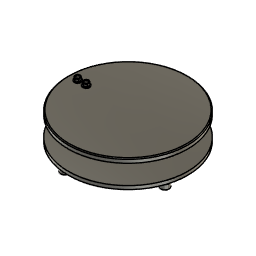
Wägezelle v2 (Autodesk Fusion 360 archive; units mm, degrees)
design "Wägezelle" references "Sechskantschraube mit Flansch und Vertiefung ANSI B18.6.7M - M4x0.7 x 16 Stahlklasse 2 Einfach", "Sechskantschraube mit Flansch und Vertiefung ANSI B18.6.7M - M4x0.7 x 20 Stahlklasse 2 Einfach"
Autodesk Fusion 360 part; units mm, degrees
note: some values were not read from the file. Chosen so that the rebuilt part matches the saved one: which bodies a step acts on; which face or edge a step refers to; how an offset face is resized. Set by a fixed rule: which sketch regions a step uses.
sketch "Skizze1" plane through (0, 0, 0) normal (0, 0, 1) x (1, 0, 0)
  line L0 (37.5, -6.35) -> (-37.5, -6.35)
  line L1 (-37.5, -6.35) -> (-37.5, 6.35)
  line L2 (-37.5, 6.35) -> (37.5, 6.35)
  line L3 (37.5, 6.35) -> (37.5, -6.35)
  line L4 (37.5, -6.35) -> (-37.5, 6.35) construction
  line L5 (-37.5, -6.35) -> (37.5, 6.35) construction
  dimension "d1" = 75
  dimension "d2" = 12.7
  constraint horizontal L0
  constraint perpendicular L0 L1
  constraint parallel L0 L2
  constraint parallel L1 L3
  constraint coincident L4 origin
  constraint coincident L5 origin
  measures "d1" distance of L1.end L2.end
  measures "d2" distance of L0.end L1.end
extrude "Extrusion1" add sketch "Skizze1" along normal blind 12.7 makes body 1
sketch "Skizze2" plane through (0, 0, 12.7) normal (0, 0, 1) x (-1, 0, 0)
  line L0 (-37.5, -6.35) -> (37.5, -6.35)
  line L1 (37.5, -6.35) -> (37.5, 6.35)
  line L2 (37.5, 6.35) -> (-37.5, 6.35)
  line L3 (-37.5, 6.35) -> (-37.5, -6.35)
  circle A0 centre (32, 0) radius 1.9
  circle A1 centre (22, 0) radius 1.9
  circle A2 centre (-32, 0) radius 1.9
  circle A3 centre (-22, 0) radius 1.9
  dimension "d8" = 3.8
  dimension "d9" = 3.8
  dimension "d10" = 5.5
  dimension "d11" = 15.5
  dimension "d12" = 3.8
  dimension "d13" = 3.8
  dimension "d14" = 5.5
  dimension "d15" = 15.5
  measures "d8" diameter of A0
  measures "d9" diameter of A1
  measures "d10" distance of L1 A0.centre
  measures "d11" distance of L1 A1.centre
  measures "d12" diameter of A2
  measures "d13" diameter of A3
  measures "d14" distance of L3 A2.centre
  measures "d15" distance of L3 A3.centre
extrude "Extrusion3" cut sketch "Skizze2" against normal through all contours A0 | A1 | A2 | A3 bodies 1
thread "Gewinde2" "ISO Metric profile 4.0 M4x0.7 6H" major diameter 4.1095 minor diameter 3.332 pitch 0.7 angle 60 resizes the face on face at (-33.8906, 0.1892, 4.2333) on bodies 1
thread "Gewinde3" "ISO Metric profile 4.0 M4x0.7 6H" major diameter 4.1095 minor diameter 3.332 pitch 0.7 angle 60 resizes the face on face at (-23.8906, 0.1892, 4.2333) on bodies 1
thread "Gewinde4" "ISO Metric profile 4.0 M4x0.7 6H" major diameter 4.1095 minor diameter 3.332 pitch 0.7 angle 60 resizes the face on face at (20.1094, 0.1892, 4.2333) on bodies 1
thread "Gewinde5" "ISO Metric profile 4.0 M4x0.7 6H" major diameter 4.1095 minor diameter 3.332 pitch 0.7 angle 60 resizes the face on face at (30.1094, 0.1892, 4.2333) on bodies 1
chamfer "Fase1" distance 0.5 angle 45 4 edges at (-37.5, 0, 12.7) (0, -6.35, 12.7) (0, 6.35, 12.7) (37.5, 0, 12.7) on bodies 1
chamfer "Fase2" distance 0.5 angle 45 1 edges at (37.5, 0, 0) 1 faces at (-7.2098, -4.7747, 0) on bodies 1
copy_body "Körper->Berechn2" bodies 1 removing the originals makes body 2 in component "Component'"
sketch "Skizze6" plane through (0, 0, 0) normal (0, 0, 1) x (1, 0, 0)
  line L0 (37, 5.85) -> (-37, 5.85)
  circle A0 centre (22, 0) radius 1.666
  circle A1 centre (32, 0) radius 1.666
  line L1 (-37, -5.85) -> (37, -5.85)
  line L2 (37, -5.85) -> (37, 5.85)
  line L3 (17.5276, 5.85) -> (37, 5.85)
  line L4 (37, 5.85) -> (37, -5.85)
  line L5 (37, -5.85) -> (17.5276, -5.85)
  line L6 (17.5276, -5.85) -> (17.5276, 5.85)
  circle A2 centre (32, 0) radius 1.9
  circle A3 centre (22, 0) radius 1.9
  dimension "d48" = 3.8
  dimension "d49" = 3.8
  constraint horizontal L3
  constraint vertical L4
  constraint horizontal L5
  constraint vertical L6
  constraint coincident L1.end L2.start
  constraint coincident L0 L3.start
  constraint concentric A1 A2
  constraint concentric A0 A3
  measures "d48" diameter of A2
  measures "d49" diameter of A3
extrude "Extrusion1'" add sketch "Skizze6" against normal blind 5 separate body contours L0 L1 L2 L3 L4 L5 L6 makes body 3 in component "Component'"
sketch "Skizze7" plane through (0, 0, -5) normal (0, 0, -1) x (1, 0, 0)
  circle A0 centre (32, 0) radius 1.9
  circle A1 centre (22, 0) radius 1.9
  line L0 (37, 5.85) -> (17.5276, 5.85)
  line L1 (17.5276, 5.85) -> (17.5276, -5.85)
  line L2 (17.5276, -5.85) -> (37, -5.85)
  line L3 (37, -5.85) -> (37, 5.85)
  circle A2 centre (26.9941, 0) radius 70
  dimension "d52" = 140
  measures "d52" diameter of A2
extrude "Extrusion2" add sketch "Skizze7" along normal blind 4 contours L0 L1 L2 L3 | A2 bodies 2 3 in component "Component'"
sketch "Skizze8" plane through (0, 0, -9) normal (0, 0, -1) x (1, 0, 0)
  circle A0 centre (32, 0) radius 1.9
  circle A1 centre (22, 0) radius 1.9
  circle A2 centre (26.9941, 0) radius 70
  circle A3 centre (42.3799, -58.7295) radius 5
  dimension "d55" = 10
  measures "d55" diameter of A3
extrude "Extrusion3'" add sketch "Skizze8" along normal blind 10 contours A3 bodies 3 in component "Component'"
fillet "Abrundung1" radius 4 1 edges at (37.7183, 56.9214, -9) on bodies 3 in component "Component'"
chamfer "Fase1'" distance 0.8 angle 45 1 edges at (37.7183, 60.5376, -19) on bodies 3 in component "Component'"
pattern_circular "C-Anordnung1" count 4 over 360 about axis through (26.9941, 0, -9) along (0, 0, -1) of "Extrusion3'" in component "Component'"
fillet "Abrundung2" radius 4 3 edges at (16.2698, -56.9214, -9) (-29.9274, 10.7242, -9) (83.9155, -10.7242, -9) on bodies 3 in component "Component'"
chamfer "Fase2'" distance 0.8 angle 45 3 edges at (87.5317, -10.7242, -19) (16.2698, -60.5376, -19) (-33.5435, 10.7242, -19) on bodies 3 in component "Component'"
sketch "Skizze9" plane through (0, 0, 12.7) normal (0, 0, 1) x (-1, 0, 0)
  circle A0 centre (32, 0) radius 1.666
  circle A1 centre (-32, 0) radius 1.666
  circle A2 centre (22, 0) radius 1.666
  circle A3 centre (-22, 0) radius 1.666
  line L0 (-37, 5.85) -> (-37, -5.85)
  line L1 (-37, -5.85) -> (37, -5.85)
  line L2 (37, -5.85) -> (37, 5.85)
  line L3 (37, 5.85) -> (-37, 5.85)
  circle A4 centre (22, 0) radius 1.666
  circle A5 centre (32, 0) radius 1.666
  line L4 (37, -5.85) -> (-37, -5.85)
  line L5 (37, 5.85) -> (37, -5.85)
  line L6 (-37, 5.85) -> (37, 5.85)
  line L7 (37, 5.85) -> (16.4735, 5.85)
  line L8 (16.4735, 5.85) -> (16.4735, -5.85)
  line L9 (16.4735, -5.85) -> (37, -5.85)
  line L10 (37, -5.85) -> (37, 5.85)
  constraint horizontal L7
  constraint vertical L8
  constraint horizontal L9
  constraint vertical L10
  constraint coincident L1 L8.end
  constraint coincident L2.end L3.start
extrude "Extrusion4" add sketch "Skizze9" along normal blind 5 separate body contours L1 L2 L3 L4 L5 L6 L7 L8 L9 L10 makes body 5 in component "Component'"
sketch "Skizze10" plane through (0, 0, 17.7) normal (0, 0, 1) x (-1, 0, 0)
  circle A0 centre (32, 0) radius 1.666
  circle A1 centre (22, 0) radius 1.666
  line L0 (37, -5.85) -> (37, 5.85)
  line L1 (37, 5.85) -> (16.4735, 5.85)
  line L2 (16.4735, 5.85) -> (16.4735, -5.85)
  line L3 (16.4735, -5.85) -> (37, -5.85)
  circle A2 centre (-26.9941, 0) radius 70
  circle A3 centre (-26.9941, 0) radius 70
  dimension "d68" = 140
  constraint concentric A2 A3
  measures "d68" diameter of A3
extrude "Extrusion4'" add sketch "Skizze10" along normal blind 5 separate body contours L0 L1 L2 L3 | A2 A3 makes body 6
other "Schraube1"
other "Schraube2"
chamfer "Fase3" distance 1 angle 45 1 edges at (92.257, 25.3131, 22.7) on bodies 6
component "Component'" placed x (1, 0, 0) y (0, 1, 0) z (0, 0, 1) at (0, 0, 0)
component "Wägezelle v2" placed x (1, 0, 0) y (0, 1, 0) z (0, 0, 1) at (0, 0, 0)
component "Wägezelle v2" placed x (1, 0, 0) y (0, 1, 0) z (0, 0, 1) at (0, 0, 0)

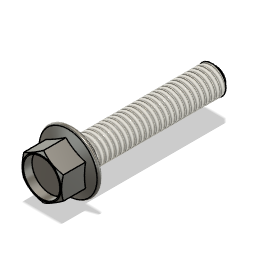
design "Sechskantschraube mit Flansch und Vertiefung ANSI B18.6.7M - M4x0.7 x 20 Stahlklasse 2 Einfach"
description: Sechskantschraube mit Flansch und Vertiefung ANSI B18.6.7M - M4x0.7 x 20
part number: IHFHMS ANSI B18.6.7M - M4x0.7 x 20 Stahlklasse 2 Einfach
Autodesk Fusion 360 part; units mm, degrees
sketch "Sketch1" plane through (0, 0, 0) normal (0, 1, 0) x (1, 0, 0)
  line L0 (-2, 0) -> (-2, 20)
  line L1 (-2, 20) -> (0, 20)
  line L2 (0, 20) -> (0, -3.1)
  line L3 (-2, 0) -> (-3.1763, 0)
  line L4 (-3.1763, 0) -> (-3.1763, -4.0222)
  line L5 (-2.695, -4.3) -> (-2.55, -4.3)
  line L6 (-2.695, -4.3) -> (-3.1763, -4.0222)
  line L7 (-2.55, -4.3) -> (-2.55, -3.1)
  line L8 (-2.55, -3.1) -> (0, -3.1)
  dimension "d9" = 4
  dimension "d111" = 4.3
  dimension "d113" = 30
  dimension "d114" = 6.3525
  dimension "d115" = 5.39
  dimension "d158" = 5.1
  dimension "d168" = 20
  dimension "d169" = 1.2
  constraint perpendicular L0 L1
  constraint perpendicular L0 L3
  constraint coincident origin L3
  constraint vertical L0
  constraint vertical L2
  constraint parallel L2 L4
  constraint coincident L2 L8.end
  constraint perpendicular L2 L5
  constraint coincident L3.end L4.start
  constraint perpendicular L5 L7
  constraint perpendicular L2 L8
  constraint coincident L2.end L8.end
  constraint coincident origin L2
  measures "d111" distance of L3 L5
  measures "d113" angle of L5 L6
  measures "d168" distance of origin L1
  measures "d169" distance of L5.end L8
revolve "Revolve1" add sketch "Sketch1" angle 360 about axis through (0, 0, -20) along (0, 0, 1)
sketch "Sketch8" plane through (0, 0, 0) normal (0, 0, 1) x (1, 0, 0)
  line L0 (0, 0) -> (-2.75, 0) construction
  line L1 (-2.75, -1.5894) -> (-2.75, 1.5894)
  circle A0 centre (0, 0) radius 3.1763
  dimension "d110" = 2.75
  constraint horizontal L0
  constraint perpendicular L0 L1
  constraint coincident L0.end L1
  constraint coincident L0.start A0.centre
  constraint coincident L1.end A0
  constraint coincident L1.start A0
  measures "d110" distance of L0.start L1
extrude "Extrude5" cut sketch "Sketch8" along normal blind 4.3 contours L1 A0 picked at (-2.8188, 0.3871)
pattern_circular "C-Pattern2" count 6 over 360 about axis through (0, 0, 1.75) along (0, 0, 1) of "Extrude5"
sketch "Sketch12" plane through (0, 0, 0) normal (0, 1, 0) x (1, 0, 0)
  line L0 (2.6125, 0) -> (3.9407, 0)
  line L1 (4.0465, -0.6) -> (2.6125, -1.1219)
  line L2 (2.6125, -1.1219) -> (2.6125, 0)
  arc A0 (4.0465, -0.6) -> (3.9407, 0) centre (3.9407, -0.3093) ccw
  line L3 (0, -1.75) -> (0, -22.5)
  line L4 (3.1763, 0) -> (3.1763, -0.9167) construction
  line L5 (0, 0) -> (2.75, 0)
  line L6 (4.25, 0) -> (4.25, -1.1219) construction
  line L7 (2.6125, -1.1219) -> (4.25, -1.1219) construction
  dimension "d122" = 5.225
  dimension "d126" = 6.3525
  dimension "d142" = 4.25
  dimension "d163" = 20
  dimension "d173" = 0.6
  constraint horizontal L0
  constraint perpendicular L0 L2
  constraint tangent L0 A0
  constraint tangent L1 A0
  constraint horizontal L5.start L0.start
  constraint coincident L1 L4.end
  constraint perpendicular L0 L4
  constraint coincident L0 L4.start
  constraint vertical L6
  constraint tangent A0 L6
  constraint coincident L0 L6.start
  constraint perpendicular L6 L7
  constraint coincident L6.end L7.end
  measures "d142" distance of L5.start L6
  measures "d163" angle of L0 L1
  measures "d173" distance of L0 L1.start
revolve "Revolve3" add sketch "Sketch12" angle 360 about axis through (0, 0, 1.75) along (0, 0, 1)
thread "Thread2" "ANSI Metric M Profile 4.0 M4x0.7 6g" major diameter 3.908 minor diameter 3.111 pitch 0.7 angle 60 resizes the face on face at (-1.9975, 0.0997, -6.6667)
fillet "Fillet4" radius 0.1333 1 edges at (1.8218, -0.7066, 0)
sketch "Sketch5" plane through (0, 0, 0) normal (0, 1, 0) x (1, 0, 0)
  line L0 (-2.04, 19.4) -> (-1.4, 20)
  line L1 (0, -1.75) -> (0, -22.5)
  line L2 (0, 20) -> (0, -3.1)
  line L3 (0, 20) -> (-2.04, 20)
  line L4 (-2.04, 20) -> (-2.04, 19.4)
  dimension "d170" = 0.6
  dimension "d171" = 1.4
  dimension "d172" = 2.04
  constraint coincident L2.start L3.start
  constraint perpendicular L2 L3
  constraint coincident L0.end L3
  constraint perpendicular L3 L4
  measures "d170" distance of L0.start L3
  measures "d171" distance of L0.end L2
  measures "d172" distance of L2.start L4
revolve "Revolve2" cut sketch "Sketch5" angle 360 about axis through (0, 0, -20) along (0, 0, 1)
equation "d9 = adsk_nomdia"
equation "adsk_nomlen = 20.00 mm"
equation "adsk_headh = 4.30 mm"
equation "adsk_nomdia = 4.00 mm"
equation "d89 = adsk_headh"
equation "adsk_waflat = 5.50 mm"
equation "d110 = adsk_waflat / 2"
equation "d111 = adsk_headh"
equation "d113 = adsk_chamang2"
equation "d114 = adsk_wacor"
equation "d115 = adsk_topdia"
equation "d122 = adsk_waflat * 0.95"
equation "d126 = adsk_waflat * 1.155"
equation "adsk_headdia = 8.50 mm"
equation "adsk_flngheig = 0.60 mm"
equation "adsk_thrlen = 18.40 mm"
equation "d133 = adsk_nomdia / 30"
equation "d142 = adsk_headdia / 2"
equation "d144 = adsk_thrlen"
equation "adsk_endpointdia = 2.80 mm"
equation "adsk_startlen = 0.60 mm"
equation "d158 = adsk_indentdia"
equation "adsk_wacor = 6.3525 mm"
equation "adsk_topdia = adsk_waflat * 0.98"
equation "adsk_chamang2 = 30.00 deg"
equation "d163 = adsk_flngang"
equation "adsk_flngang = 20.00 deg"
equation "adsk_indentdia = 5.10 mm"
equation "adsk_indentdepth = 1.20 mm"
equation "d168 = adsk_nomlen"
equation "d169 = adsk_indentdepth"
equation "d170 = adsk_startlen"
equation "d171 = adsk_endpointdia / 2"
equation "d172 = adsk_nomdia * 0.51"
equation "d173 = adsk_flngheig"

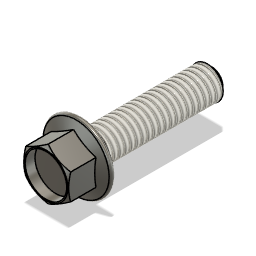
design "Sechskantschraube mit Flansch und Vertiefung ANSI B18.6.7M - M4x0.7 x 16 Stahlklasse 2 Einfach"
description: Sechskantschraube mit Flansch und Vertiefung ANSI B18.6.7M - M4x0.7 x 16
part number: IHFHMS ANSI B18.6.7M - M4x0.7 x 16 Stahlklasse 2 Einfach
Autodesk Fusion 360 part; units mm, degrees
sketch "Sketch1" plane through (0, 0, 0) normal (0, 1, 0) x (1, 0, 0)
  line L0 (-2, 0) -> (-2, 16)
  line L1 (-2, 16) -> (0, 16)
  line L2 (0, 16) -> (0, -3.1)
  line L3 (-2, 0) -> (-3.1763, 0)
  line L4 (-3.1763, 0) -> (-3.1763, -4.0222)
  line L5 (-2.695, -4.3) -> (-2.55, -4.3)
  line L6 (-2.695, -4.3) -> (-3.1763, -4.0222)
  line L7 (-2.55, -4.3) -> (-2.55, -3.1)
  line L8 (-2.55, -3.1) -> (0, -3.1)
  dimension "d9" = 4
  dimension "d111" = 4.3
  dimension "d113" = 30
  dimension "d114" = 6.3525
  dimension "d115" = 5.39
  dimension "d158" = 5.1
  dimension "d168" = 16
  dimension "d169" = 1.2
  constraint perpendicular L0 L1
  constraint perpendicular L0 L3
  constraint coincident origin L3
  constraint vertical L0
  constraint vertical L2
  constraint parallel L2 L4
  constraint coincident L2 L8.end
  constraint perpendicular L2 L5
  constraint coincident L3.end L4.start
  constraint perpendicular L5 L7
  constraint perpendicular L2 L8
  constraint coincident L2.end L8.end
  constraint coincident origin L2
  measures "d111" distance of L3 L5
  measures "d113" angle of L5 L6
  measures "d168" distance of origin L1
  measures "d169" distance of L5.end L8
revolve "Revolve1" add sketch "Sketch1" angle 360 about axis through (0, 0, -16) along (0, 0, 1)
sketch "Sketch8" plane through (0, 0, 0) normal (0, 0, 1) x (1, 0, 0)
  line L0 (0, 0) -> (-2.75, 0) construction
  line L1 (-2.75, -1.5894) -> (-2.75, 1.5894)
  circle A0 centre (0, 0) radius 3.1763
  dimension "d110" = 2.75
  constraint horizontal L0
  constraint perpendicular L0 L1
  constraint coincident L0.end L1
  constraint coincident L0.start A0.centre
  constraint coincident L1.end A0
  constraint coincident L1.start A0
  measures "d110" distance of L0.start L1
extrude "Extrude5" cut sketch "Sketch8" along normal blind 4.3 contours L1 A0 picked at (-2.8188, -0.3871)
pattern_circular "C-Pattern2" count 6 over 360 about axis through (0, 0, 1.75) along (0, 0, 1) of "Extrude5"
sketch "Sketch12" plane through (0, 0, 0) normal (0, 1, 0) x (1, 0, 0)
  line L0 (2.6125, 0) -> (3.9407, 0)
  line L1 (4.0465, -0.6) -> (2.6125, -1.1219)
  line L2 (2.6125, -1.1219) -> (2.6125, 0)
  arc A0 (4.0465, -0.6) -> (3.9407, 0) centre (3.9407, -0.3093) ccw
  line L3 (0, -1.75) -> (0, -22.5)
  line L4 (3.1763, 0) -> (3.1763, -0.9167) construction
  line L5 (0, 0) -> (2.75, 0)
  line L6 (4.25, 0) -> (4.25, -1.1219) construction
  line L7 (2.6125, -1.1219) -> (4.25, -1.1219) construction
  dimension "d122" = 5.225
  dimension "d126" = 6.3525
  dimension "d142" = 4.25
  dimension "d163" = 20
  dimension "d173" = 0.6
  constraint horizontal L0
  constraint perpendicular L0 L2
  constraint tangent L0 A0
  constraint tangent L1 A0
  constraint horizontal L5.start L0.start
  constraint coincident L1 L4.end
  constraint perpendicular L0 L4
  constraint coincident L0 L4.start
  constraint vertical L6
  constraint tangent A0 L6
  constraint coincident L0 L6.start
  constraint perpendicular L6 L7
  constraint coincident L6.end L7.end
  measures "d142" distance of L5.start L6
  measures "d163" angle of L0 L1
  measures "d173" distance of L0 L1.start
revolve "Revolve3" add sketch "Sketch12" angle 360 about axis through (0, 0, 1.75) along (0, 0, 1)
thread "Thread2" "ANSI Metric M Profile 4.0 M4x0.7 6g" major diameter 3.908 minor diameter 3.111 pitch 0.7 angle 60 resizes the face on face at (-1.9975, 0.0997, -5.3333)
fillet "Fillet4" radius 0.1333 1 edges at (1.8218, -0.7066, 0)
sketch "Sketch5" plane through (0, 0, 0) normal (0, 1, 0) x (1, 0, 0)
  line L0 (-2.04, 15.4) -> (-1.4, 16)
  line L1 (0, -1.75) -> (0, -22.5)
  line L2 (0, 16) -> (0, -3.1)
  line L3 (0, 16) -> (-2.04, 16)
  line L4 (-2.04, 16) -> (-2.04, 15.4)
  dimension "d170" = 0.6
  dimension "d171" = 1.4
  dimension "d172" = 2.04
  constraint coincident L2.start L3.start
  constraint perpendicular L2 L3
  constraint coincident L0.end L3
  constraint perpendicular L3 L4
  measures "d170" distance of L0.start L3
  measures "d171" distance of L0.end L2
  measures "d172" distance of L2.start L4
revolve "Revolve2" cut sketch "Sketch5" angle 360 about axis through (0, 0, -16) along (0, 0, 1)
equation "d9 = adsk_nomdia"
equation "adsk_nomlen = 16.00 mm"
equation "adsk_headh = 4.30 mm"
equation "adsk_nomdia = 4.00 mm"
equation "d89 = adsk_headh"
equation "adsk_waflat = 5.50 mm"
equation "d110 = adsk_waflat / 2"
equation "d111 = adsk_headh"
equation "d113 = adsk_chamang2"
equation "d114 = adsk_wacor"
equation "d115 = adsk_topdia"
equation "d122 = adsk_waflat * 0.95"
equation "d126 = adsk_waflat * 1.155"
equation "adsk_headdia = 8.50 mm"
equation "adsk_flngheig = 0.60 mm"
equation "adsk_thrlen = 14.40 mm"
equation "d133 = adsk_nomdia / 30"
equation "d142 = adsk_headdia / 2"
equation "d144 = adsk_thrlen"
equation "adsk_endpointdia = 2.80 mm"
equation "adsk_startlen = 0.60 mm"
equation "d158 = adsk_indentdia"
equation "adsk_wacor = 6.3525 mm"
equation "adsk_topdia = adsk_waflat * 0.98"
equation "adsk_chamang2 = 30.00 deg"
equation "d163 = adsk_flngang"
equation "adsk_flngang = 20.00 deg"
equation "adsk_indentdia = 5.10 mm"
equation "adsk_indentdepth = 1.20 mm"
equation "d168 = adsk_nomlen"
equation "d169 = adsk_indentdepth"
equation "d170 = adsk_startlen"
equation "d171 = adsk_endpointdia / 2"
equation "d172 = adsk_nomdia * 0.51"
equation "d173 = adsk_flngheig"
